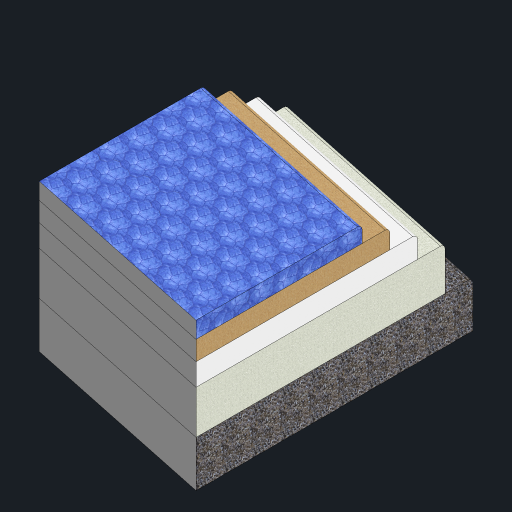
# Autodesk Inventor part: 부품1
Saved by Autodesk Inventor 2024.1 (Build 281209000, 209)
## iProperties
Created: 2024-01-19
Part Number: 부품1
Material: 일반
Document SubType Name: Modeling
Designer: KBU
Density: 1 g/cm^3
Appearance: 기본값
Author: KBU
Autodesk Inventor part; units mm, degrees
ref_plane "YZ Plane" through (0, 0, 0) normal (1, 0, 0) x (0, 1, 0)
ref_plane "XZ Plane" through (0, 0, 0) normal (0, 1, 0) x (-1, 0, 0)
ref_plane "XY Plane" through (0, 0, 0) normal (0, 0, 1) x (1, 0, 0)
sketch "스케치8" plane through (0, 0, 0) normal (0, 0, 1) x (1, 0, 0)
  line L0 (0, 0) -> (0, 250)
  line L1 (0, 250) -> (-850, 477.7568)
  line L2 (-850, 477.7568) -> (-850, 227.7568)
  line L3 (-850, 227.7568) -> (0, 0)
  line L4 (-40.1649, 0) -> (36.8005, 0)
  line L5 (-850, 477.7568) -> (-850, 1027.7568)
  line L6 (-850, 1027.7568) -> (0, 800)
  line L7 (0, 800) -> (0, 250)
  line L8 (-850, 712.7568) -> (0, 485)
  line L9 (0, 605) -> (-850, 832.7568)
  line L10 (-850, 937.7568) -> (0, 710)
  dimension "d23" = 15
  dimension "d24" = 850
  dimension "d25" = 800
  dimension "d26" = 235
  dimension "d27" = 120
  dimension "d28" = 105
  dimension "d40" = 250
  dimension "d46" = 90
  constraints: 22 end point, 7 parallel, 6 point on line, 2 horizontal, 2 vertical
  measures "d23" angle of L3 L4
  measures "d24" distance between parallel lines of L0 L2
  measures "d25" distance of L2.end L5.end
  measures "d26" distance of L1.end L8.start
  measures "d27" distance of L9.end L8.start
  measures "d28" distance of L10.start L9.end
  measures "d40" distance of L1.end L2.end
  measures "d46" distance of L5.end L10.start
extrude "돌출9" add sketch "스케치8" against normal blind 1500 contours L3 L2 L1 L0
extrude "돌출10" add sketch "스케치8" against normal blind 1350 separate body contours L1 L5 L8 L7
extrude "돌출11" add sketch "스케치8" against normal blind 1200 separate body contours L8 L5 L9 L7
extrude "돌출12" add sketch "스케치8" against normal blind 1050 separate body contours L9 L5 L10 L7
extrude "돌출13" add sketch "스케치8" against normal blind 900 separate body contours L10 L5 L6 L7
fillet "모깎기2" radius 25 5 edges at (-425, 363.8784, -1500) (-425, 598.8784, -1350) (-425, 718.8784, -1200) (-425, 823.8784, -1050) (-425, 913.8784, -900)
